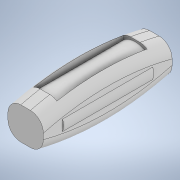
# Autodesk Inventor part: Weapon-Healing-Stock
Saved by Autodesk Inventor 2020 (Build 240168000, 168)
## iProperties
Created: 2019-12-04
Part Number: Weapon-Healing-Stock
Material: Generic
Document SubType Name: Modeling
Designer: vifly_01
Density: 1 g/cm^3
Appearance: Default
Author: vifly_01
Autodesk Inventor part; units mm, degrees
ref_plane "YZ Plane" through (0, 0, 0) normal (1, 0, 0) x (0, 1, 0)
ref_plane "XZ Plane" through (0, 0, 0) normal (0, 1, 0) x (-1, 0, 0)
ref_plane "XY Plane" through (0, 0, 0) normal (0, 0, 1) x (1, 0, 0)
sketch "Sketch1" plane through (0, 0, 0) normal (0, 0, 1) x (1, 0, 0)
  line L0 (5.5, -7.5) -> (-5.5, -7.5)
  line L1 (-5.5, -7.5) -> (-5.5, 7.5)
  line L2 (-5.5, 7.5) -> (5.5, 7.5)
  line L3 (5.5, 7.5) -> (5.5, -7.5)
  line L4 (5.5, -7.5) -> (-5.5, 7.5) construction
  line L5 (-5.5, -7.5) -> (5.5, 7.5) construction
  point P0 (0, 0)
  dimension "d0" = 11
  dimension "d1" = 15
  constraints: 12 end point, 2 midpoint, 2 parallel, 1 horizontal, 1 perpendicular
  measures "d0" distance of L1.end L2.end
  measures "d1" distance of L0.end L1.end
extrude "Extrusion1" add sketch "Sketch1" along normal blind 40
sketch "Sketch2" plane through (5.5, -7.5, 0) normal (1, 0, 0) x (0, 0, -1)
  line L0 (0, 15) -> (-40, 15) projected
  line L1 (-20, 11.6201) -> (0, 11.6201) construction
  line L2 (-20, 11.6201) -> (0, 11.6201) construction
  line L3 (-20, 2.5) -> (0, 2.5) construction
  line L4 (-20, 2.5) -> (0, 2.5) construction
  line L5 (-40, 15) -> (-20, 15)
  line L6 (-20, 15) -> (0, 15)
  line L7 (0, 2.5) -> (0, 0)
  line L8 (0, 0) -> (-20, 0)
  line L9 (0, 0) -> (-40, 0) projected
  line L10 (-20, 0) -> (-40, 0)
  line L11 (0, 0) -> (0, 15) projected
  line L12 (-40, 0) -> (-40, 15) projected
  arc A0 (0, 12.5) -> (-40, 12.5) centre (-20, -66.25) ccw
  line L13 (-40, 12.5) -> (0, 12.5) construction
  line L14 (-40, 12.5) -> (0, 12.5) construction
  line L15 (-40, 12.5) -> (-40, 15)
  line L16 (0, 12.5) -> (0, 15)
  arc A1 (-40, 2.5) -> (0, 2.5) centre (-20, 81.25) ccw
  line L17 (0, 0) -> (-40, 0) projected
  line L18 (-40, 2.5) -> (-40, 0)
  line L19 (-20, 0) -> (-40, 0)
  line L20 (-20, 0) -> (0, 0)
  point P0 (0, 7.5)
  dimension "d4" = 0
  dimension "d5" = 0
  dimension "d9" = 2.5
  dimension "d10" = 0
  constraints: 32 end point, 5 collinear, 5 point on circle, 4 horizontal, 3 tangent, 2 centre point, 2 midpoint, 2 vertical, 1 point on line, 3 other
  measures "d4" distance between parallel lines of L1 L2
  measures "d5" distance between parallel lines of L3 L4
  measures "d9" distance of L7.end L3.end
  measures "d10" distance between parallel lines of L13 L14
extrude "Extrusion3" cut sketch "Sketch2" against normal blind 12 contours L11 A0 L0 | A0 L12 L0 | L7 L8 A1 | A1 L9 L12
fillet "Fillet2" radius 4 4 edges at (5.5, 7.5, 20) (5.5, -7.5, 20) (-5.5, 7.5, 20) (-5.5, -7.5, 20)
ref_plane "Work Plane1" through (0, 0, 20) normal (0, 0, 1) x (1, 0, 0)
sketch "Sketch10" plane through (0, 0, 0) normal (0, 1, 0) x (-1, 0, 0)
  line L0 (3.462, 34) -> (-3.7054, 34)
  line L1 (-3.7054, 34) -> (-3.7054, 6)
  line L2 (-3.7054, 6) -> (3.462, 6)
  line L3 (3.462, 6) -> (3.462, 34)
  point P0 (0, 0)
  constraints: 8 end point, 2 parallel, 1 horizontal, 1 perpendicular
extrude "Extrusion5" cut sketch "Sketch10" along normal blind 28
sketch "Sketch9" plane through (0, 0, 20) normal (0, 0, 1) x (1, 0, 0)
  circle A0 centre (0, 0) radius 5.75
  dimension "d24" = 11.5
  constraints: 1 centre point, 1 coincident
  measures "d24" diameter of A0
extrude "Extrusion4" add sketch "Sketch9" along normal mid plane 28
body "Solid1"
